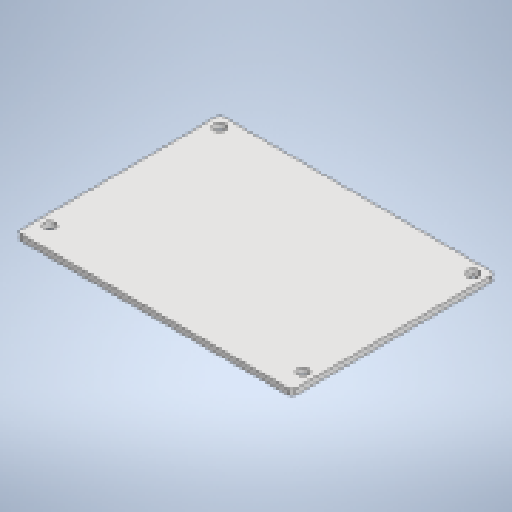
# Autodesk Inventor part: pcb_glowne
Saved by Autodesk Inventor 2023 (Build 270158000, 158)
## iProperties
Created: 2024-04-28
Part Number: pcb_glowne
Material: Ogólny
Document SubType Name: Modeling
Designer: kamil
Density: 1 g/cm^3
Appearance: Domyślna
Author: kamil
Autodesk Inventor part; units mm, degrees
ref_plane "YZ Plane" through (0, 0, 0) normal (1, 0, 0) x (0, 1, 0)
ref_plane "XZ Plane" through (0, 0, 0) normal (0, 1, 0) x (-1, 0, 0)
ref_plane "XY Plane" through (0, 0, 0) normal (0, 0, 1) x (1, 0, 0)
sketch "Szkic1" plane through (0, 0, 0) normal (0, 1, 0) x (-1, 0, 0)
  line L0 (24.7544, 40.9723) -> (-51.2456, 40.9723)
  line L1 (-51.2456, 40.9723) -> (-51.2456, -15.1007)
  line L2 (-51.2456, -15.1007) -> (24.7544, -15.1007)
  line L3 (24.7544, -15.1007) -> (24.7544, 40.9723)
  point P0 (0, 0)
  dimension "d0" = 76
  dimension "d1" = 56.073
  constraints: 8 end point, 2 parallel, 1 horizontal, 1 perpendicular
  measures "d0" distance of L0.start L0.end
  measures "d1" distance of L2.end L0.start
extrude "Wyciągnięcie proste1" add sketch "Szkic1" along normal blind 1.6
fillet "Zaokrąglenie1" radius 1 4 edges at (51.2456, 0.8, -15.1007) (51.2456, 0.8, 40.9723) (-24.7544, 0.8, 40.9723) (-24.7544, 0.8, -15.1007)
sketch "Szkic2" plane through (0, 1.6, 0) normal (0, 1, 0) x (1, 0, 0)
  circle A0 centre (-21.7544, 12.1007) radius 1.6 projected
  circle A1 centre (48.2456, 12.1007) radius 1.6 projected
  circle A2 centre (-21.7544, -34.9723) radius 1.6 projected
  circle A3 centre (48.2456, -34.9723) radius 1.6 projected
  point P0 (0, 0)
  constraints: 4 coincident
hole "Otwór1" at (-21.7544, 1.6, -12.1007) at (48.2456, 1.6, -12.1007) at (-21.7544, 1.6, 34.9723) at (48.2456, 1.6, 34.9723) direction (0, -1, 0) diameter 3 end through all
